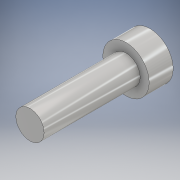
# Autodesk Inventor part: M2_SCREW_8MM
Saved by Autodesk Inventor 2017.3 (Build 213256000, 256)
## iProperties
Created: 2018-01-04
Part Number: M2_SCREW_8MM
Material: Generic
Document SubType Name: Modeling
Designer: Alex
Density: 1 g/cm^3
Appearance: Aluminum - Polished
Author: Alex
Autodesk Inventor part; units mm, degrees
ref_plane "YZ Plane" through (0, 0, 0) normal (1, 0, 0) x (0, 1, 0)
ref_plane "XZ Plane" through (0, 0, 0) normal (0, 1, 0) x (-1, 0, 0)
ref_plane "XY Plane" through (0, 0, 0) normal (0, 0, 1) x (1, 0, 0)
sketch "Sketch1" plane through (0, 0, 0) normal (0, 1, 0) x (-1, 0, 0)
  circle A0 centre (0, 0) radius 1.175
  dimension "d0" = 2.35
  constraints: 1 centre point, 1 coincident
  measures "d0" diameter of A0
extrude "Extrusion1" add sketch "Sketch1" along normal blind 8
sketch "Sketch2" plane through (0, 8, 0) normal (0, 1, 0) x (1, 0, 0)
  circle A0 centre (0, 0) radius 1.175 projected
  circle A1 centre (0, 0) radius 1.925
  dimension "d3" = 3.85
  constraints: 1 centre point, 1 coincident
  measures "d3" diameter of A1
extrude "Extrusion2" add sketch "Sketch2" along normal blind 2 contours A0 | A1
sketch "Sketch3" plane through (0, 10, 0) normal (0, 1, 0) x (1, 0, 0)
  line L0 (-0.4961, 0.7099) -> (0.3667, 0.7845)
  line L1 (0.3667, 0.7845) -> (0.8628, 0.0747)
  line L2 (0.8628, 0.0747) -> (0.4961, -0.7099)
  line L3 (0.4961, -0.7099) -> (-0.3667, -0.7845)
  line L4 (-0.3667, -0.7845) -> (-0.8628, -0.0747)
  line L5 (-0.8628, -0.0747) -> (-0.4961, 0.7099)
  point P0 (0, 0)
  point P1 (0, 0)
  dimension "d6" = 1.5
  constraints: 12 end point, 1 coincident, 13 other
  measures "d6" distance between parallel lines of L0 L3
extrude "Extrusion3" cut sketch "Sketch3" against normal blind 1
body "Solid1"
